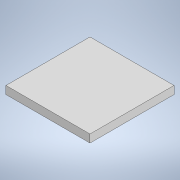
# Autodesk Inventor part: woodForkSupportBase
Saved by Autodesk Inventor 2021 (Build 250183000, 183)
## iProperties
Created: 2020-07-02
Part Number: woodForkSupportBase
Material: Generic
Document SubType Name: Modeling
Designer: robst
Density: 1 g/cm^3
Appearance: Default
Author: robst
Autodesk Inventor part; units mm, degrees
ref_plane "YZ Plane" through (0, 0, 0) normal (1, 0, 0) x (0, 1, 0)
ref_plane "XZ Plane" through (0, 0, 0) normal (0, 1, 0) x (-1, 0, 0)
ref_plane "XY Plane" through (0, 0, 0) normal (0, 0, 1) x (1, 0, 0)
sketch "Sketch1" plane through (0, 0, 0) normal (0, 1, 0) x (-1, 0, 0)
  line L0 (101.6, 101.6) -> (-101.6, 101.6)
  line L1 (-101.6, 101.6) -> (-101.6, -101.6)
  line L2 (-101.6, -101.6) -> (101.6, -101.6)
  line L3 (101.6, -101.6) -> (101.6, 101.6)
  line L4 (101.6, 101.6) -> (-101.6, -101.6) construction
  line L5 (-101.6, 101.6) -> (101.6, -101.6) construction
  point P0 (0, 0)
  dimension "d0" = 203.2
  dimension "d1" = 203.2
  constraints: 12 end point, 2 midpoint, 2 parallel, 1 horizontal, 1 perpendicular
  measures "d0" distance of L2.end L0.start
  measures "d1" distance of L0.start L0.end
extrude "Extrusion1" add sketch "Sketch1" against normal blind 19.05
body "Solid1"
